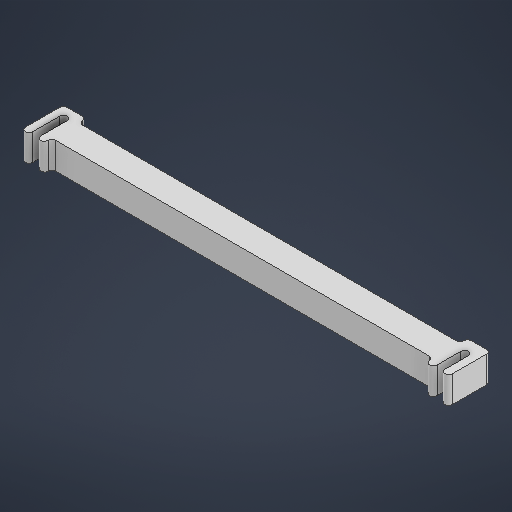
# Autodesk Inventor part: rozpěrka
Saved by Autodesk Inventor 2026.1 (Build 301233000, 233)
## iProperties
Created: 2026-01-08
Part Number: rozpěrka
Material: Všeobecné
Document SubType Name: Modeling
Designer: bubli
Density: 1 g/cm^3
Appearance: Výchozí
Author: bubli
Autodesk Inventor part; units mm, degrees
ref_plane "YZ Plane" through (0, 0, 0) normal (1, 0, 0) x (0, 1, 0)
ref_plane "XZ Plane" through (0, 0, 0) normal (0, 1, 0) x (-1, 0, 0)
ref_plane "XY Plane" through (0, 0, 0) normal (0, 0, 1) x (1, 0, 0)
sketch "Náčrt1" plane through (0, 0, 0) normal (0, 0, 1) x (1, 0, 0)
  line L0 (-46.6467, 2.3751) -> (53.3533, 2.3751)
  line L1 (53.3533, 2.3751) -> (53.3533, -4.6249)
  line L2 (53.3533, -4.6249) -> (-46.6467, -4.6249)
  line L3 (-46.6467, -4.6249) -> (-46.6467, 2.3751)
  line L4 (-46.6467, 4.3751) -> (-52.6467, 4.3751)
  line L5 (-52.6467, 4.3751) -> (-52.6467, -6.6249)
  line L6 (-46.6467, -6.6249) -> (-46.6467, 4.3751)
  line L7 (-50.6467, 2.3751) -> (-48.6467, 2.3751)
  line L8 (-48.6467, 2.3751) -> (-48.6467, -6.6249)
  line L9 (-50.6467, -6.6249) -> (-50.6467, 2.3751)
  line L10 (-52.6467, -6.6249) -> (-50.6467, -6.6249)
  line L11 (-48.6467, -6.6249) -> (-46.6467, -6.6249)
  line L12 (53.3533, 4.3751) -> (59.3533, 4.3751)
  line L13 (59.3533, 4.3751) -> (59.3533, -6.6249)
  line L14 (53.3533, -6.6249) -> (53.3533, 4.3751)
  line L15 (57.3533, -6.6249) -> (57.3533, 1.5943)
  line L16 (57.3533, 1.5943) -> (55.3533, 1.5943)
  line L17 (55.3533, 1.5943) -> (55.3533, -6.6249)
  line L18 (59.3533, -6.6249) -> (57.3533, -6.6249)
  line L19 (55.3533, -6.6249) -> (53.3533, -6.6249)
  point P0 (0, 0)
  point P1 (-47.6467, -6.6249)
  point P2 (56.3533, 4.3751)
  point P3 (55.3533, -2.5153)
  point P4 (54.3533, -6.6249)
  dimension "d0" = 100
  dimension "d1" = 7
  dimension "d2" = 2
  dimension "d4" = 6
  dimension "d5" = 2
  dimension "d6" = 0
  dimension "d7" = 2
  dimension "d8" = 2
  dimension "d9" = 2
  dimension "d10" = 2
  dimension "d11" = 6
  dimension "d12" = 0
  dimension "d14" = 2
  dimension "d15" = 2
  dimension "d16" = 2
  constraints: 40 end point, 10 parallel, 4 horizontal, 4 midpoint, 4 perpendicular, 1 point on line
  measures "d0" distance of L0.start L0.end
  measures "d1" distance of L2.end L0.start
  measures "d2" distance between parallel lines of L0 L4
  measures "d4" distance between parallel lines of L6 L5
  measures "d5" distance between parallel lines of L8 L9
  measures "d6" distance between parallel lines of L0 L7
  measures "d7" distance from line of L2 point (-47.647, -6.625)
  measures "d8" distance between parallel lines of L2 L10
  measures "d9" distance between parallel lines of L3 L8
  measures "d10" distance from line of L0 point (56.353, 4.375)
  measures "d11" distance between parallel lines of L13 L1
  measures "d12" distance between parallel lines of L1 L14
  measures "d14" distance from line of point (55.353, -2.515) L1
  measures "d15" distance between parallel lines of L15 L17
  measures "d16" distance from line of point (54.353, -6.625) L2
extrude "Vysunutí1" add sketch "Náčrt1" along normal blind 7
fillet "Zaoblení1" radius 1 3 edges at (-46.6467, 4.3751, 3.5) (-46.6467, 2.3751, 3.5) (-52.6467, 4.3751, 3.5)
fillet "Zaoblení2" radius 1 3 edges at (53.3533, 2.3751, 3.5) (53.3533, 4.3751, 3.5) (59.3533, 4.3751, 3.5)
fillet "Zaoblení3" radius 1 5 edges at (-46.6467, -4.6249, 3.5) (-46.6467, -6.6249, 3.5) (-48.6467, -6.6249, 3.5) (-50.6467, -6.6249, 3.5) (-52.6467, -6.6249, 3.5)
fillet "Zaoblení4" radius 1 5 edges at (53.3533, -6.6249, 3.5) (53.3533, -4.6249, 3.5) (55.3533, -6.6249, 3.5) (57.3533, -6.6249, 3.5) (59.3533, -6.6249, 3.5)
fillet "Zaoblení5" radius 1 4 edges at (-50.6467, 2.3751, 3.5) (-48.6467, 2.3751, 3.5) (55.3533, 1.5943, 3.5) (57.3533, 1.5943, 3.5)
